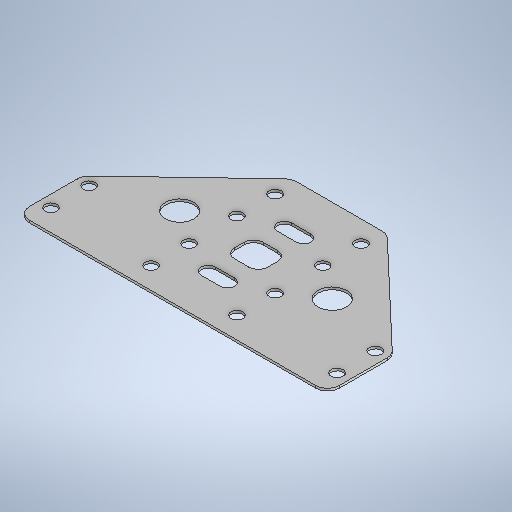
# Autodesk Inventor part: 16
Saved by Autodesk Inventor 2025.1 (Build 291241000, 241)
## iProperties
Created: 2024-09-13
Part Number: 16
Material: Generisch
Document SubType Name: Modeling
Designer: ffogue
Density: 1 g/cm^3
Appearance: Vorgabe
Author: ffogue
Autodesk Inventor part; units mm, degrees
ref_plane "YZ Plane" through (0, 0, 0) normal (1, 0, 0) x (0, 1, 0)
ref_plane "XZ Plane" through (0, 0, 0) normal (0, 1, 0) x (-1, 0, 0)
sketch "Sketch1" plane through (0, 0, 0) normal (0, 0, 1) x (1, 0, 0)
  line L0 (-32.5, 0) -> (32.5, 0)
  line L1 (32.5, 0) -> (32.5, 13.6)
  line L2 (32.5, 13.6) -> (10, 35)
  line L3 (10, 35) -> (-10, 35)
  line L4 (-10, 35) -> (-32.5, 13.6)
  line L5 (-32.5, 13.6) -> (-32.5, 0)
  line L6 (0, 0) -> (0, 41.5771) construction
  dimension "d0" = 13.6
  dimension "d1" = 65
  dimension "d2" = 35
  dimension "d3" = 20
  constraints: 14 end point, 3 symmetric about line, 2 parallel, 1 horizontal, 1 midpoint, 1 perpendicular, 1 vertical
  measures "d0" distance of L4.end L0.start
  measures "d1" distance of L0.start L0.end
  measures "d2" distance between parallel lines of L0 L3
  measures "d3" distance of L2.end L3.end
extrude "Extrusion1" add sketch "Sketch1" along normal blind 0.5
fillet "Fillet1" radius 2.5 4 edges at (-32.5, 13.6, 0.25) (32.5, 13.6, 0.25) (10, 35, 0.25) (-10, 35, 0.25)
sketch "Sketch2" plane through (0, 0, 0.5) normal (0, 0, 1) x (1, 0, 0)
  arc A0 (-9.001, 35) -> (-10.7239, 34.3115) centre (-9.001, 32.5) ccw projected
  line L0 (9.001, 35) -> (-9.001, 35) projected
  line L1 (-32.5, 0) -> (32.5, 0) projected
  point P0 (0, 0)
  point P1 (0, 35)
  point P2 (-30, 12.5)
  point P3 (30, 12.5)
  point P4 (30, 4.5)
  point P5 (-30, 4.5)
  point P6 (0, 0)
  point P7 (-16, 17.5)
  point P8 (16, 17.5)
  point P9 (0, 35)
  dimension "d9" = 60
  dimension "d10" = 30
  dimension "d11" = 4.5
  dimension "d12" = 8
  dimension "d13" = 16
  dimension "d14" = 32
  dimension "d15" = 5
  constraints: 3 horizontal alignment, 3 midpoint, 2 vertical alignment
  measures "d9" distance of point (30, 4.5) point (-30, 4.5)
  measures "d10" horizontal distance of point (0, 0) point (-30, 4.5)
  measures "d11" distance from line of L1 point (-30, 4.5)
  measures "d12" distance of point (-30, 4.5) point (-30, 12.5)
  measures "d13" horizontal distance of point (0, 35) point (-16, 17.5)
  measures "d14" distance of point (16, 17.5) point (-16, 17.5)
  measures "d15" vertical distance of point (-30, 12.5) point (-16, 17.5)
hole "Hole1" at (-16, 17.5, 0.5) at (16, 17.5, 0.5) direction (0, 0, -1) diameter 6 depth 0.5
hole "Hole2" at (-30, 12.5, 0.5) at (30, 12.5, 0.5) at (30, 4.5, 0.5) at (-30, 4.5, 0.5) direction (0, 0, -1) diameter 2.5 depth 0.5
sketch "Sketch3" plane through (0, 0, 0) normal (0, 0, -1) x (-1, 0, 0)
  line L0 (-3.5, 14.5) -> (3.5, 14.5)
  line L1 (3.5, 14.5) -> (3.5, 20.5)
  line L2 (3.5, 20.5) -> (-3.5, 20.5)
  line L3 (-3.5, 20.5) -> (-3.5, 14.5)
  line L4 (-3.5, 14.5) -> (3.5, 20.5) construction
  line L5 (3.5, 14.5) -> (-3.5, 20.5) construction
  circle A0 centre (-16, 17.5) radius 3 projected
  line L6 (32.5, 0) -> (-32.5, 0) projected
  point P0 (0, 0)
  point P1 (0, 17.5)
  point P2 (-3.5, 17.5)
  point P3 (0, 0)
  dimension "d30" = 7
  dimension "d31" = 6
  constraints: 12 end point, 4 midpoint, 2 parallel, 1 horizontal, 1 horizontal alignment, 1 perpendicular, 1 vertical alignment
  measures "d30" distance of L1.end L2.end
  measures "d31" distance of L2.end L0.start
extrude "Extrusion2" cut sketch "Sketch3" against normal up to surface (0.5 mm away) contours L3 L2 L1 L0
fillet "Fillet2" radius 2 4 edges at (3.5, 20.5, 0.25) (-3.5, 20.5, 0.25) (-3.5, 14.5, 0.25) (3.5, 14.5, 0.25)
sketch "Sketch4" plane through (0, 0, 0) normal (0, 0, -1) x (-1, 0, 0)
  line L0 (-2, 9.5) -> (2, 9.5) construction
  line L1 (-2, 11) -> (2, 11)
  line L2 (2, 8) -> (-2, 8)
  arc A0 (-2, 11) -> (-2, 8) centre (-2, 9.5) ccw
  arc A1 (2, 8) -> (2, 11) centre (2, 9.5) ccw
  line L3 (32.5, 0) -> (-32.5, 0) projected
  circle A2 centre (30, 12.5) radius 1.25 projected
  point P0 (0, 0)
  point P1 (0, 9.5)
  point P2 (0, 0)
  point P3 (0, 0)
  point P4 (0, 0)
  point P5 (0, 0)
  dimension "d35" = 1.5
  dimension "d37" = 4
  dimension "d39" = 3
  dimension "d40" = 2
  constraints: 8 end point, 5 midpoint, 4 point on circle, 4 tangent, 3 vertical alignment, 2 centre point, 1 parallel
  measures "d35" radius of A0
  measures "d37" distance of L0.start L0.end
  measures "d39" distance from line of L0 A2.centre
  measures "d40" horizontal distance of point (0, 0) L0.end
extrude "Extrusion3" cut sketch "Sketch4" against normal up to surface (0.5 mm away) contours L1 A1 L2 A0
ref_plane "Work Plane1" through (-9.001, 17.5, 0) normal (0, 1, 0) x (1, 0, 0)
mirror "Mirror1" about plane through (-9.001, 17.5, 0) normal (0, 1, 0) of "Extrusion3"
sketch "Sketch5" plane through (0, 0, 0) normal (0, 0, -1) x (-1, 0, 0)
  circle A0 centre (-30, 12.5) radius 1.25 projected
  line L0 (32.5, 0) -> (-32.5, 0) projected
  point P0 (0, 0)
  point P1 (-9, 12.5)
  point P2 (9, 12.5)
  point P3 (0, 0)
  point P4 (-9, 4.5)
  point P5 (9, 4.5)
  dimension "d44" = 18
  dimension "d45" = 9
  dimension "d46" = 4.5
  constraints: 3 horizontal alignment, 2 vertical alignment, 1 midpoint
  measures "d44" distance of point (9, 12.5) point (-9, 12.5)
  measures "d45" horizontal distance of point (0, 0) point (-9, 12.5)
  measures "d46" distance from line of L0 point (-9, 4.5)
hole "Hole3" at (9, 12.5, 0) at (-9, 12.5, 0) at (9, 4.5, 0) at (-9, 4.5, 0) direction (0, 0, 1) diameter 2.5 depth 0.5
mirror "Mirror2" about plane through (-9.001, 17.5, 0) normal (0, 1, 0) of "Hole3"
fillet "Fillet3" radius 2.5 2 edges at (-32.5, 0, 0.25) (32.5, 0, 0.25)
equation "\"d10\" = 0.5 * d9"
equation "\"d45\" = 0.5 * d44"
body "Solid1"
